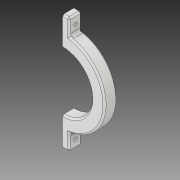
# Autodesk Inventor part: 2122_Copper Tube Clamp Top_V1
Saved by Autodesk Inventor 2020 (Build 240168000, 168)
## iProperties
Created: 2017-06-29
Part Number: 2122_Copper Tube Clamp Top_V1
Material: ABS Plastic
Document SubType Name: Modeling
Designer: MPI
Density: 1.06 g/cm^3
Appearance: Smooth - White
Mass: 174.205 g
Surface Area: 290.765 cm^2
Volume: 164.344 cm^3
Author: MPI
Autodesk Inventor part; units mm, degrees
ref_plane "YZ Plane" through (0, 0, 0) normal (1, 0, 0) x (0, 1, 0)
ref_plane "XZ Plane" through (0, 0, 0) normal (0, 1, 0) x (-1, 0, 0)
ref_plane "XY Plane" through (0, 0, 0) normal (0, 0, 1) x (1, 0, 0)
sketch "Sketch1" plane through (0, 0, 0) normal (0, 0, 1) x (1, 0, 0)
  circle A0 centre (0, 0) radius 56.515
  line L0 (12.7, -114.3) -> (-12.7, -114.3)
  line L1 (-12.7, 114.3) -> (12.7, 114.3)
  line L2 (12.7, 114.3) -> (-12.7, -114.3) construction
  line L3 (12.7, -114.3) -> (-12.7, 114.3) construction
  line L4 (12.7, -81.5672) -> (12.7, -114.3)
  line L5 (-12.7, -114.3) -> (-12.7, -81.5672)
  line L6 (12.7, 114.3) -> (12.7, 81.5672)
  arc A1 (12.7, -81.5672) -> (12.7, 81.5672) centre (0, 0) ccw
  arc A2 (-12.7, 81.5672) -> (-12.7, -81.5672) centre (0, 0) ccw
  line L7 (-12.7, 81.5672) -> (-12.7, 114.3)
  line L8 (0, 114.3) -> (0, -114.3)
  line L9 (-0.7937, -114.3) -> (0.7937, -114.3)
  line L10 (0.7937, -114.3) -> (0.7937, 114.3)
  line L11 (0.7937, 114.3) -> (-0.7937, 114.3)
  line L12 (-0.7937, 114.3) -> (-0.7937, -114.3)
  line L13 (-0.7937, -114.3) -> (0.7937, 114.3) construction
  line L14 (0.7937, -114.3) -> (-0.7937, 114.3) construction
  dimension "d0" = 113.03
  dimension "d1" = 228.6
  dimension "d2" = 25.4
  dimension "d3" = 82.55
  dimension "d4" = 82.55
  dimension "d5" = 32.7328
  dimension "d6" = 32.7328
  dimension "d7" = 1.5875
  constraints: 30 end point, 7 parallel, 6 midpoint, 4 point on circle, 3 centre point, 3 perpendicular, 2 vertical, 1 coincident, 1 horizontal, 1 point on line
  measures "d0" diameter of A0
  measures "d1" distance of L1.end L0.start
  measures "d2" distance of L0.start L0.end
  measures "d3" radius of A1
  measures "d4" radius of A2
  measures "d5" distance of L7.start L1.start
  measures "d6" distance of L1.end L6.end
  measures "d7" distance of L11.end L10.end
extrude "Extrusion1" add sketch "Sketch1" along normal blind 25.4 contours A0 L10 | A0 L10 L1 L6 A1 L4 L0 | L10 A0 L8 | A0 L8 L1 L10 | L10 L0 L8 A0
sketch "Sketch2" plane through (0, 0, 25.4) normal (0, 0, 1) x (1, 0, 0)
  arc A0 (12.7, -81.5672) -> (12.7, 81.5672) centre (0, 0) ccw projected
  circle A1 centre (0, 0) radius 56.515
  dimension "d10" = 113.03
  constraints: 1 centre point, 1 coincident
  measures "d10" diameter of A1
extrude "Extrusion2" cut sketch "Sketch2" against normal blind 25.4
sketch "Sketch3" plane through (12.7, 81.5672, 0) normal (1, 0, 0) x (0, 0, -1)
  line L0 (-25.4, 32.7328) -> (0, 0) construction
  line L1 (0, -138.0822) -> (0, -195.8672) projected
  line L2 (-25.4, -163.1345) -> (0, -195.8672) construction
  point P0 (0, -81.5672)
  point P1 (-12.7, -179.5008)
  point P2 (-12.7, 16.3664)
  constraints: 4 end point, 2 midpoint, 1 coincident
hole "Hole1" at (12.7, -97.9336, 12.7) at (12.7, 97.9336, 12.7) direction (-1, 0, 0) diameter 6.858 depth 15.6718 tip angle 118 clearance for "Flat Head Machine Screw (82)" size "1/4" standard "Ansi Unified Screw Threads"
chamfer "Chamfer1" distance 3.175 angle 45 14 edges at (56.515, 0, 25.4) (56.515, 0, 0) (82.55, 0, 0) (82.55, 0, 25.4) (12.7, 97.9336, 25.4) (12.7, 114.3, 12.7) (12.7, 97.9336, 0) (12.7, -97.9336, 0) (12.7, -97.9336, 25.4) (12.7, -114.3, 12.7) (6.35, -114.3, 25.4) (6.35, -114.3, 0) (6.35, 114.3, 25.4) (6.35, 114.3, 0)
fillet "Fillet1" radius 6.35 2 edges at (12.7, -81.5672, 12.7) (12.7, 81.5672, 12.7)
equation "\"d4\" = d3"
equation "\"d6\" = d5"
body "Solid1"
